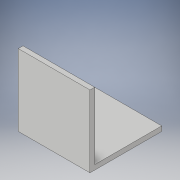
# Autodesk Inventor part: Winkel
Saved by Autodesk Inventor 2017.3 (Build 213256000, 256)
## iProperties
Part Number: Winkel
Material: Generisch
Document SubType Name: Modeling
Designer: Nils
Density: 1 g/cm^3
Appearance: Vorgabe
Author: Nils
Autodesk Inventor part; units mm, degrees
ref_plane "YZ Plane" through (0, 0, 0) normal (1, 0, 0) x (0, 1, 0)
ref_plane "XZ Plane" through (0, 0, 0) normal (0, 1, 0) x (-1, 0, 0)
ref_plane "XY Plane" through (0, 0, 0) normal (0, 0, 1) x (1, 0, 0)
sketch "Skizze1" plane through (0, 0, 0) normal (1, 0, 0) x (0, 1, 0)
  line L0 (-12.2718, -10.7427) -> (15.7282, -10.7427)
  line L1 (15.7282, -10.7427) -> (15.7282, -12.7427)
  line L2 (15.7282, -12.7427) -> (-14.2718, -12.7427)
  line L3 (-14.2718, -12.7427) -> (-14.2718, 3.7136)
  line L4 (-14.2718, -12.7427) -> (-6.9903, -12.7427)
  line L5 (-12.2718, -10.7427) -> (-12.2718, 17.2573)
  line L6 (-12.2718, 17.2573) -> (-14.2718, 17.2573)
  line L7 (-14.2718, 17.2573) -> (-14.2718, -12.7427)
  point P0 (0, 0)
  dimension "d0" = 30
  dimension "d1" = 30
  dimension "d2" = 2
  dimension "d3" = 2
  constraints: 16 end point, 4 parallel, 2 horizontal, 2 perpendicular
  measures "d0" distance of L1.end L2.end
  measures "d1" distance of L6.end L2.end
  measures "d2" distance of L0.end L1.end
  measures "d3" distance of L5.end L6.end
extrude "Extrusion1" add sketch "Skizze1" along normal mid plane 30
